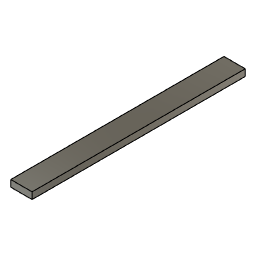
Assembly (no drawer) (Autodesk Fusion 360 archive; units mm, degrees)
design "Rail (2x)"
Autodesk Fusion 360 part; units mm, degrees
sketch "Sketch1" plane through (0, 0, 0) normal (0, 0, 1) x (1, 0, 0)
  line L0 (0, 0) -> (10.16, 0)
  line L1 (10.16, 0) -> (10.16, 101.6)
  line L2 (10.16, 101.6) -> (0, 101.6)
  line L3 (0, 101.6) -> (0, 0)
  dimension "d1" = 10.16
  dimension "d2" = 101.6
  constraint coincident L0.start L3.end
  constraint horizontal L0
  constraint perpendicular L0 L1
  constraint perpendicular L1 L2
  constraint perpendicular L0 L3
  measures "d1" distance of L0.start L0.end
  measures "d2" distance of L0.end L1.end
extrude "Extrude1" add sketch "Sketch1" along normal blind 3.175

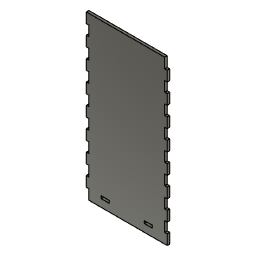
design "Dice Tower (Back)"
Autodesk Fusion 360 part; units mm, degrees
sketch "Sketch1" plane through (0, 0, 0) normal (0, 1, 0) x (1, 0, 0)
  line L0 (3.175, -50.8) -> (3.175, -38.1)
  line L1 (3.175, -38.1) -> (3.175, -25.4)
  line L2 (6.35, -12.7) -> (3.175, -12.7)
  line L3 (3.175, -63.5) -> (6.35, -63.5)
  line L4 (3.175, -76.2) -> (3.175, -63.5)
  line L5 (6.35, -25.4) -> (3.175, -25.4)
  line L6 (3.175, -88.9) -> (3.175, -76.2)
  line L7 (6.35, -25.4) -> (6.35, -38.1)
  line L8 (6.35, -38.1) -> (3.175, -38.1)
  line L9 (3.175, -12.7) -> (3.175, 0)
  line L10 (3.175, -60.2676) -> (2.1543, -60.2676)
  line L11 (3.175, 0) -> (3.175, -59.055)
  line L12 (6.35, 0) -> (3.175, 0)
  line L13 (3.175, -25.4) -> (3.175, -12.7)
  line L14 (3.175, -101.6) -> (3.175, -88.9)
  line L15 (3.175, -76.2) -> (6.35, -76.2)
  line L16 (-95.25, -25.4) -> (-95.25, -12.7)
  line L17 (-92.075, -139.7) -> (-95.25, -139.7)
  line L18 (3.175, 0) -> (3.175, -203.2)
  line L19 (-92.075, -50.8) -> (-95.25, -50.8)
  line L20 (3.175, -50.8) -> (6.35, -50.8)
  line L21 (6.35, 0) -> (-4.7498, 0)
  line L22 (3.175, -88.9) -> (6.35, -88.9)
  line L23 (-92.075, -38.1) -> (-92.075, -25.4)
  line L24 (-92.075, -127) -> (-92.075, -114.3)
  line L25 (-95.25, 0) -> (6.35, 0)
  line L26 (-92.075, -203.2) -> (-92.075, -190.5)
  line L27 (3.175, -63.5) -> (3.175, -50.8)
  line L28 (6.35, -50.8) -> (6.35, -63.5)
  line L29 (-92.075, 0) -> (-92.075, -203.2)
  line L30 (6.35, -76.2) -> (6.35, -88.9)
  line L31 (-92.075, -95.25) -> (-92.075, -88.9)
  line L32 (6.35, 0) -> (-5.715, 0)
  line L33 (-95.25, 0) -> (-79.375, 0)
  line L34 (-92.075, -25.4) -> (-95.25, -25.4)
  line L35 (-92.075, -76.2) -> (-92.075, -63.5)
  line L36 (-4.7498, 0) -> (0.3302, 0)
  line L37 (6.35, 0) -> (6.35, -12.7)
  line L38 (6.35, -101.6) -> (3.175, -101.6)
  line L39 (-92.075, -177.8) -> (-95.25, -177.8)
  line L40 (-84.1502, 0) -> (-89.2302, 0)
  line L41 (-92.075, -139.7) -> (-92.075, -127)
  line L42 (-89.5189, -92.8088) -> (-89.7576, -92.8956)
  line L43 (-95.25, -101.6) -> (-95.25, -88.9)
  line L44 (6.35, -177.8) -> (6.35, -190.5)
  line L45 (6.35, -152.4) -> (6.35, -165.1)
  line L46 (3.175, -203.2) -> (3.175, -190.5)
  line L47 (3.175, -190.5) -> (3.175, -177.8)
  line L48 (-92.075, -63.5) -> (-95.25, -63.5)
  line L49 (-92.075, -25.4) -> (-92.075, -12.7)
  line L50 (-92.075, -190.5) -> (-95.25, -190.5)
  line L51 (-92.075, -12.7) -> (-95.25, -12.7)
  line L52 (3.175, -203.2) -> (-95.25, -203.2)
  line L53 (-92.075, -177.8) -> (-92.075, -165.1)
  line L54 (-92.075, -101.6) -> (-92.075, -95.25)
  line L55 (-92.075, -76.2) -> (-95.25, -76.2)
  line L56 (-95.25, -76.2) -> (-95.25, -63.5)
  line L57 (3.175, -114.3) -> (6.35, -114.3)
  line L58 (-95.25, -203.2) -> (-95.25, -190.5)
  line L59 (-92.075, -63.5) -> (-92.075, -50.8)
  line L60 (-92.075, -50.8) -> (-92.075, -38.1)
  line L61 (-92.075, -152.4) -> (-95.25, -152.4)
  line L62 (-92.075, -88.9) -> (-95.25, -88.9)
  line L63 (-92.075, -152.4) -> (-92.075, -139.7)
  line L64 (-95.25, -203.2) -> (-92.075, -203.2)
  line L65 (6.35, -152.4) -> (3.175, -152.4)
  line L66 (-92.075, -165.1) -> (-92.075, -152.4)
  line L67 (-92.075, -203.2) -> (-92.075, -177.8)
  line L68 (-92.075, -165.1) -> (-95.25, -165.1)
  line L69 (-92.075, -114.3) -> (-95.25, -114.3)
  line L70 (6.35, -101.6) -> (6.35, -114.3)
  line L71 (-95.25, -127) -> (-95.25, -114.3)
  line L72 (-92.075, -114.3) -> (-92.075, -101.6)
  line L73 (6.35, -139.7) -> (6.35, -127)
  line L74 (6.35, -127) -> (6.35, -139.7)
  line L75 (3.175, -177.8) -> (6.35, -177.8)
  line L76 (3.175, -165.1) -> (6.35, -165.1)
  line L77 (-92.075, -38.1) -> (-95.25, -38.1)
  line L78 (6.35, -114.3) -> (6.35, -101.6)
  line L79 (-95.25, 0) -> (-84.1502, 0)
  line L80 (-92.075, -127) -> (-95.25, -127)
  line L81 (3.175, -152.4) -> (3.175, -139.7)
  line L82 (-95.25, -177.8) -> (-95.25, -165.1)
  line L83 (6.35, -165.1) -> (6.35, -152.4)
  line L84 (-92.075, -101.6) -> (-95.25, -101.6)
  line L85 (3.175, -139.7) -> (6.35, -139.7)
  line L86 (-95.25, 0) -> (-92.075, 0)
  line L87 (-95.25, -152.4) -> (-95.25, -139.7)
  line L88 (3.175, -127) -> (3.175, -114.3)
  line L89 (6.35, -127) -> (3.175, -127)
  line L90 (3.175, -190.5) -> (6.35, -190.5)
  line L91 (-92.075, -88.9) -> (-92.075, -76.2)
  line L92 (-95.25, 0) -> (-93.6625, 0)
  line L93 (-92.075, -190.5) -> (-92.075, -177.8)
  line L94 (3.175, -177.8) -> (3.175, -165.1)
  line L95 (-95.25, -50.8) -> (-95.25, -38.1)
  point P0 (6.35, 0)
  point P1 (6.35, 0)
  dimension "d9" = 11.0998
  dimension "d10" = 11.0998
  dimension "d14" = 5.08
  dimension "d15" = 5.08
  dimension "d27" = 3.175
  dimension "d28" = 3.175
  dimension "d40" = 3.175
  dimension "d41" = 3.175
  dimension "d42" = 12.7
  dimension "d43" = 12.7
  dimension "d44" = 12.7
  dimension "d45" = 12.7
  dimension "d46" = 12.7
  dimension "d47" = 12.7
  dimension "d48" = 12.7
  dimension "d49" = 12.7
  dimension "d50" = 6.35
  dimension "d52" = 12.7
  dimension "d53" = 12.7
  dimension "d54" = 12.7
  dimension "d55" = 12.7
  dimension "d56" = 12.7
  dimension "d57" = 12.7
  constraint coincident P1 P0
  constraint perpendicular L37 L52
  constraint perpendicular L52 L58
  constraint perpendicular L25 L37
  constraint perpendicular L32 L37
  constraint perpendicular L33 L58
  constraint perpendicular L58 L92
  constraint coincident L40.start L25
  constraint perpendicular L21 L37
  constraint perpendicular L37 L90
  constraint perpendicular L47 L90
  constraint coincident L44.start L37
  constraint perpendicular L37 L75
  constraint perpendicular L75 L94
  constraint perpendicular L37 L76
  constraint collinear L37 L44
  constraint perpendicular L76 L83
  constraint perpendicular L65 L83
  constraint parallel L12 L32
  constraint perpendicular L18 L52
  constraint perpendicular L65 L81
  constraint coincident L88.start L18
  constraint perpendicular L18 L89
  constraint perpendicular L88 L89
  constraint perpendicular L57 L88
  constraint perpendicular L18 L38
  constraint perpendicular L14 L38
  constraint parallel L0 L1
  constraint parallel L13 L18
  constraint coincident L15.end L37
  constraint coincident L20.end L37
  constraint coincident L5.start L37
  constraint collinear L37 L45
  constraint collinear L37 L74
  constraint collinear L37 L70
  constraint collinear L30 L37
  constraint collinear L28 L37
  constraint collinear L7 L37
  constraint perpendicular L58 L64
  constraint perpendicular L58 L86
  constraint perpendicular L26 L52
  constraint perpendicular L50 L58
  constraint perpendicular L50 L93
  constraint coincident L39.end L58
  constraint perpendicular L39 L58
  constraint perpendicular L39 L53
  constraint coincident L68.end L58
  constraint perpendicular L58 L68
  constraint perpendicular L66 L68
  constraint coincident L61.end L58
  constraint perpendicular L58 L61
  constraint perpendicular L61 L63
  constraint coincident L17.end L58
  constraint perpendicular L17 L58
  constraint perpendicular L17 L41
  constraint coincident L71.start L58
  constraint perpendicular L58 L80
  constraint perpendicular L24 L80
  constraint coincident L69.end L58
  constraint perpendicular L58 L69
  constraint perpendicular L69 L72
  constraint perpendicular L58 L84
  constraint perpendicular L54 L84
  constraint parallel L29 L31
  constraint coincident L43.end L58
  constraint perpendicular L58 L62
  constraint perpendicular L62 L91
  constraint coincident L55.end L58
  constraint perpendicular L55 L58
  constraint perpendicular L35 L55
  constraint coincident L48.end L58
  constraint perpendicular L48 L58
  constraint perpendicular L48 L59
  constraint coincident L19.end L58
  constraint perpendicular L19 L58
  constraint perpendicular L19 L60
  constraint coincident L77.end L58
  constraint perpendicular L58 L77
  constraint perpendicular L23 L77
  constraint perpendicular L23 L34
  constraint perpendicular L34 L49
  constraint perpendicular L49 L51
  constraint collinear L58 L82
  constraint coincident L43.start L58
  constraint collinear L82 L87
  constraint collinear L71 L87
  constraint collinear L43 L71
  constraint collinear L43 L56
  constraint collinear L56 L95
  constraint collinear L16 L95
  constraint coincident L11.end L27
  constraint coincident L10.start L27
  measures "d9" distance of L40.start L25.start
  measures "d10" distance of P1 L21.end
  measures "d14" distance of L36.end L21.end
  measures "d15" distance of L40.start L40.end
  measures "d27" distance of L65.end L45.start
  measures "d28" distance of P1 L9.end
  measures "d40" distance of L52.end L26.start
  measures "d41" distance of L25.start L29.start
  measures "d42" distance of L26.end L26.start
  measures "d43" distance of L39.start L26.end
  measures "d44" distance of L39.start L53.end
  measures "d45" distance of L61.start L53.end
  measures "d46" distance of L61.start L17.start
  measures "d47" distance of L24.start L17.start
  measures "d48" distance of L24.start L24.end
  measures "d49" distance of L54.start L24.end
  measures "d50" distance of L54.start L31.start
  measures "d52" distance of L35.start L31.end
  measures "d53" distance of L35.start L35.end
  measures "d54" distance of L19.start L35.end
  measures "d55" distance of L23.start L19.start
  measures "d56" distance of L23.end L23.start
  measures "d57" distance of L49.end L23.end
extrude "Extrude1" add sketch "Sketch1" along normal blind 3.175
sketch "Sketch2" plane through (0, 0, 0) normal (0, -1, 0) x (1, 0, 0)
  line L0 (-95.25, 63.5) -> (-92.075, 63.5)
  line L1 (-92.075, 63.5) -> (-92.075, 50.8)
  line L2 (-92.075, 50.8) -> (-95.25, 50.8)
  line L3 (-95.25, 50.8) -> (-95.25, 38.1)
  line L4 (-95.25, 38.1) -> (-92.075, 38.1)
  line L5 (-92.075, 38.1) -> (-92.075, 25.4)
  line L6 (-92.075, 25.4) -> (-95.25, 25.4)
  line L7 (-95.25, 25.4) -> (-95.25, 12.7)
  line L8 (-95.25, 12.7) -> (-92.075, 12.7)
  line L9 (-92.075, 12.7) -> (-92.075, 0)
  line L10 (-92.075, 0) -> (6.35, 0)
  line L11 (6.35, 0) -> (6.35, 12.7)
  line L12 (6.35, 12.7) -> (3.175, 12.7)
  line L13 (3.175, 12.7) -> (3.175, 25.4)
  line L14 (3.175, 25.4) -> (6.35, 25.4)
  line L15 (6.35, 25.4) -> (6.35, 38.1)
  line L16 (6.35, 38.1) -> (3.175, 38.1)
  line L17 (3.175, 38.1) -> (3.175, 50.8)
  line L18 (3.175, 50.8) -> (6.35, 50.8)
  line L19 (6.35, 50.8) -> (6.35, 63.5)
  line L20 (6.35, 63.5) -> (3.175, 63.5)
  line L21 (3.175, 63.5) -> (3.175, 76.2)
  line L22 (3.175, 76.2) -> (6.35, 76.2)
  line L23 (6.35, 76.2) -> (6.35, 88.9)
  line L24 (6.35, 88.9) -> (3.175, 88.9)
  line L25 (3.175, 88.9) -> (3.175, 101.6)
  line L26 (3.175, 101.6) -> (6.35, 101.6)
  line L27 (6.35, 101.6) -> (6.35, 114.3)
  line L28 (6.35, 114.3) -> (3.175, 114.3)
  line L29 (3.175, 114.3) -> (3.175, 127)
  line L30 (3.175, 127) -> (6.35, 127)
  line L31 (6.35, 127) -> (6.35, 139.7)
  line L32 (6.35, 139.7) -> (3.175, 139.7)
  line L33 (3.175, 139.7) -> (3.175, 152.4)
  line L34 (3.175, 152.4) -> (6.35, 152.4)
  line L35 (6.35, 152.4) -> (6.35, 165.1)
  line L36 (6.35, 165.1) -> (3.175, 165.1)
  line L37 (3.175, 165.1) -> (3.175, 177.8)
  line L38 (3.175, 177.8) -> (6.35, 177.8)
  line L39 (6.35, 177.8) -> (6.35, 190.5)
  line L40 (6.35, 190.5) -> (3.175, 190.5)
  line L41 (3.175, 190.5) -> (3.175, 203.2)
  line L42 (3.175, 203.2) -> (-95.25, 203.2)
  line L43 (-95.25, 203.2) -> (-95.25, 190.5)
  line L44 (-95.25, 190.5) -> (-92.075, 190.5)
  line L45 (-92.075, 190.5) -> (-92.075, 177.8)
  line L46 (-92.075, 177.8) -> (-95.25, 177.8)
  line L47 (-95.25, 177.8) -> (-95.25, 165.1)
  line L48 (-95.25, 165.1) -> (-92.075, 165.1)
  line L49 (-92.075, 165.1) -> (-92.075, 152.4)
  line L50 (-92.075, 152.4) -> (-95.25, 152.4)
  line L51 (-95.25, 152.4) -> (-95.25, 139.7)
  line L52 (-95.25, 139.7) -> (-92.075, 139.7)
  line L53 (-92.075, 139.7) -> (-92.075, 127)
  line L54 (-92.075, 127) -> (-95.25, 127)
  line L55 (-95.25, 127) -> (-95.25, 114.3)
  line L56 (-95.25, 114.3) -> (-92.075, 114.3)
  line L57 (-92.075, 114.3) -> (-92.075, 101.6)
  line L58 (-92.075, 101.6) -> (-95.25, 101.6)
  line L59 (-95.25, 101.6) -> (-95.25, 88.9)
  line L60 (-95.25, 88.9) -> (-92.075, 88.9)
  line L61 (-92.075, 88.9) -> (-92.075, 76.2)
  line L62 (-92.075, 76.2) -> (-95.25, 76.2)
  line L63 (-95.25, 76.2) -> (-95.25, 63.5)
  line L64 (6.35, 0) -> (-12.3698, 0)
  line L65 (-12.3698, 0) -> (-12.3698, 9.525)
  line L66 (-92.075, 0) -> (-76.5302, 0)
  line L67 (-76.5302, 0) -> (-76.5302, 9.525)
  line L68 (-76.5302, 9.525) -> (-66.3702, 9.525)
  line L69 (-66.3702, 9.525) -> (-66.3702, 12.7)
  line L70 (-66.3702, 12.7) -> (-76.5302, 12.7)
  line L71 (-76.5302, 12.7) -> (-76.5302, 9.525)
  line L72 (-12.3698, 9.525) -> (-22.5298, 9.525)
  line L73 (-22.5298, 9.525) -> (-22.5298, 12.7)
  line L74 (-22.5298, 12.7) -> (-12.3698, 12.7)
  line L75 (-12.3698, 12.7) -> (-12.3698, 9.525)
  dimension "d105" = 18.7198
  dimension "d106" = 9.525
  dimension "d107" = 15.5448
  dimension "d108" = 9.525
  dimension "d109" = 10.16
  dimension "d110" = 3.175
  dimension "d111" = 10.16
  dimension "d112" = 10.16
  dimension "d113" = 10.16
  constraint coincident L10.end L11.start
  constraint perpendicular L11 L64
  constraint perpendicular L64 L65
  constraint coincident L9.end L10.start
  constraint perpendicular L9 L66
  constraint perpendicular L66 L67
  constraint perpendicular L67 L68
  constraint perpendicular L68 L69
  constraint perpendicular L69 L70
  constraint perpendicular L65 L72
  constraint perpendicular L72 L73
  constraint perpendicular L73 L74
  measures "d105" distance of L10.end L64.end
  measures "d106" distance of L64.end L65.end
  measures "d107" distance of L9.end L66.end
  measures "d108" distance of L66.end L67.end
  measures "d109" distance of L67.end L68.end
  measures "d110" distance of L68.end L69.end
  measures "d111" distance of L69.end L70.end
  measures "d112" distance of L65.end L72.end
  measures "d113" distance of L73.end L74.end
extrude "Extrude2" cut sketch "Sketch2" against normal blind 20.32 contours L68 L69 L70 L71 | L72 L73 L74 L75
equation "d9 = 0.5 in - 0.063 in"

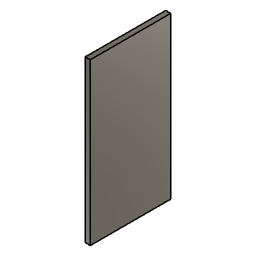
design "Ramp (Top Ramp x2)"
Autodesk Fusion 360 part; units mm, degrees
sketch "Sketch1" plane through (0, 0, 0) normal (1, 0, 0) x (0, 1, 0)
  line L0 (0, 0) -> (50.8, 0)
  line L1 (50.8, 0) -> (50.8, 101.6)
  line L2 (50.8, 101.6) -> (0, 101.6)
  line L3 (0, 101.6) -> (0, 0)
  dimension "d1" = 50.8
  dimension "d2" = 101.6
  constraint coincident L0.start L3.end
  constraint horizontal L0
  constraint perpendicular L0 L1
  constraint perpendicular L1 L2
  constraint perpendicular L2 L3
  measures "d1" distance of L0.start L0.end
  measures "d2" distance of L0.end L1.end
extrude "Extrude1" add sketch "Sketch1" along normal blind 3.175

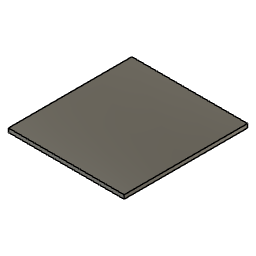
design "Ramp (Bottem Ramp 1x)"
Autodesk Fusion 360 part; units mm, degrees
sketch "Sketch1" plane through (0, 0, 0) normal (0, 0, 1) x (1, 0, 0)
  line L0 (0, 0) -> (95.25, 0)
  line L1 (95.25, 0) -> (95.25, 101.6)
  line L2 (95.25, 101.6) -> (0, 101.6)
  line L3 (0, 101.6) -> (0, 0)
  dimension "d1" = 95.25
  dimension "d2" = 101.6
  dimension "d3" = 95.25
  constraint coincident L0.start L3.end
  constraint horizontal L0
  constraint perpendicular L0 L1
  constraint perpendicular L1 L2
  measures "d1" distance of L0.start L0.end
  measures "d2" distance of L0.end L1.end
  measures "d3" distance of L1.end L2.end
extrude "Extrude1" add sketch "Sketch1" along normal blind 3.175

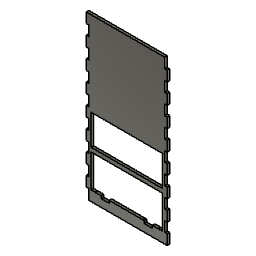
design "Dice Tower (FRONT)"
Autodesk Fusion 360 part; units mm, degrees
sketch "Sketch2" plane through (0, 0, 0) normal (0, 0, 1) x (1, 0, 0)
sketch "Sketch3" plane through (0, 0, 0) normal (0, 1, 0) x (1, 0, 0)
  line L0 (85.725, 0) -> (101.6, 0)
  line L1 (88.9, -50.8) -> (85.725, -50.8)
  line L2 (187.325, -12.7) -> (184.15, -12.7)
  line L3 (104.4448, -12.7) -> (104.4448, -9.525)
  line L4 (88.9, -12.7) -> (85.725, -12.7)
  line L5 (85.725, -25.4) -> (85.725, -12.7)
  line L6 (91.7448, -12.7) -> (104.4448, -12.7)
  line L7 (88.9, -63.5) -> (88.9, -50.8)
  line L8 (181.3052, -12.7) -> (168.6052, -12.7)
  line L9 (88.9, -76.2) -> (88.9, -63.5)
  line L10 (181.3052, -53.975) -> (91.7448, -53.975)
  line L11 (85.725, 0) -> (87.3125, 0)
  line L12 (91.7448, 0) -> (91.7448, -12.7)
  line L13 (88.9, -50.8) -> (88.9, -38.1)
  line L14 (88.9, -25.4) -> (88.9, -12.7)
  line L15 (176.2252, 0) -> (181.3052, 0)
  line L16 (187.325, -38.1) -> (184.15, -38.1)
  line L17 (158.4452, -12.7) -> (156.5402, -12.7)
  line L18 (96.8248, -12.7) -> (104.4448, -12.7)
  line L19 (168.6052, -12.7) -> (176.2252, -12.7)
  line L20 (91.7448, -12.7) -> (96.8248, -12.7)
  line L21 (88.9, -38.1) -> (88.9, -25.4)
  line L22 (168.6052, -12.7) -> (168.6052, -9.525)
  line L23 (96.8248, 0) -> (91.7448, 0)
  line L24 (187.325, -25.4) -> (184.15, -25.4)
  line L25 (88.9, -25.4) -> (85.725, -25.4)
  line L26 (114.6048, -12.7) -> (156.5402, -12.7)
  line L27 (158.4452, -9.525) -> (158.4452, -12.7)
  line L28 (114.6048, -9.525) -> (114.6048, -12.7)
  line L29 (187.325, 0) -> (187.325, -12.7)
  line L30 (181.3052, -12.7) -> (176.2252, -12.7)
  line L31 (187.325, 0) -> (184.15, 0)
  line L32 (85.725, 0) -> (96.8248, 0)
  line L33 (187.325, 0) -> (176.2252, 0)
  line L34 (184.15, -12.7) -> (184.15, 0)
  line L35 (184.15, -25.4) -> (184.15, -12.7)
  line L36 (88.9, -139.7) -> (85.725, -139.7)
  line L37 (88.9, -101.6) -> (88.9, -95.25)
  line L38 (88.9, -127) -> (85.725, -127)
  line L39 (88.9, -95.25) -> (88.9, -88.9)
  line L40 (184.15, -101.6) -> (184.15, -88.9)
  line L41 (88.9, -114.3) -> (88.9, -101.6)
  line L42 (187.325, -101.6) -> (187.325, -114.3)
  line L43 (184.15, -127) -> (184.15, -114.3)
  line L44 (88.9, -127) -> (88.9, -114.3)
  line L45 (187.325, -101.6) -> (184.15, -101.6)
  line L46 (187.325, -139.7) -> (187.325, -127)
  line L47 (184.15, -139.7) -> (187.325, -139.7)
  line L48 (88.9, -114.3) -> (85.725, -114.3)
  line L49 (88.9, -139.7) -> (88.9, -127)
  line L50 (187.325, -114.3) -> (187.325, -101.6)
  line L51 (187.325, -127) -> (184.15, -127)
  line L52 (88.9, -88.9) -> (85.725, -88.9)
  line L53 (91.7448, -97.155) -> (181.3052, -97.155)
  line L54 (85.725, -101.6) -> (85.725, -88.9)
  line L55 (88.9, -101.6) -> (85.725, -101.6)
  line L56 (187.325, -127) -> (187.325, -139.7)
  line L57 (184.15, -88.9) -> (187.325, -88.9)
  line L58 (184.15, -114.3) -> (187.325, -114.3)
  line L59 (85.725, -127) -> (85.725, -114.3)
  line L60 (184.15, 0) -> (184.15, -203.2)
  line L61 (85.725, -203.2) -> (88.9, -203.2)
  line L62 (88.9, 0) -> (88.9, -203.2)
  line L63 (88.9, -165.1) -> (88.9, -152.4)
  line L64 (187.325, -152.4) -> (187.325, -165.1)
  line L65 (184.15, -203.2) -> (184.15, -190.5)
  line L66 (184.15, -152.4) -> (184.15, -139.7)
  line L67 (88.9, -203.2) -> (88.9, -190.5)
  line L68 (85.725, -152.4) -> (85.725, -139.7)
  line L69 (88.9, -165.1) -> (85.725, -165.1)
  line L70 (88.9, -190.5) -> (85.725, -190.5)
  line L71 (88.9, -177.8) -> (85.725, -177.8)
  line L72 (184.15, -177.8) -> (187.325, -177.8)
  line L73 (184.15, -190.5) -> (184.15, -177.8)
  line L74 (88.9, -152.4) -> (88.9, -139.7)
  line L75 (184.15, -165.1) -> (187.325, -165.1)
  line L76 (187.325, -177.8) -> (187.325, -190.5)
  line L77 (88.9, -152.4) -> (85.725, -152.4)
  line L78 (187.325, -152.4) -> (184.15, -152.4)
  line L79 (184.15, -190.5) -> (187.325, -190.5)
  line L80 (184.15, -76.2) -> (187.325, -76.2)
  line L81 (181.3052, 0) -> (181.3052, -12.7)
  line L82 (91.7448, -59.055) -> (181.3052, -59.055)
  line L83 (187.325, -165.1) -> (187.325, -152.4)
  line L84 (91.7448, -59.055) -> (91.7448, -97.155)
  line L85 (88.9, -63.5) -> (85.725, -63.5)
  line L86 (184.15, -177.8) -> (184.15, -165.1)
  line L87 (184.15, -50.8) -> (184.15, -38.1)
  line L88 (85.725, 0) -> (187.325, 0)
  line L89 (184.15, -63.5) -> (187.325, -63.5)
  line L90 (187.325, -25.4) -> (187.325, -38.1)
  line L91 (187.325, 0) -> (175.26, 0)
  line L92 (184.15, -76.2) -> (184.15, -63.5)
  line L93 (181.3052, -59.055) -> (181.3052, -97.155)
  line L94 (187.325, -50.8) -> (187.325, -63.5)
  line L95 (168.6052, -9.525) -> (158.4452, -9.525)
  line L96 (184.15, -38.1) -> (184.15, -25.4)
  line L97 (85.725, -76.2) -> (85.725, -63.5)
  line L98 (85.725, -177.8) -> (85.725, -165.1)
  line L99 (91.7448, -12.7) -> (91.7448, -53.975)
  line L100 (85.725, -50.8) -> (85.725, -38.1)
  line L101 (104.4448, -9.525) -> (114.6048, -9.525)
  line L102 (184.15, -50.8) -> (187.325, -50.8)
  line L103 (88.9, -177.8) -> (88.9, -165.1)
  line L104 (181.3052, -12.7) -> (181.3052, -53.975)
  line L105 (187.325, -76.2) -> (187.325, -88.9)
  line L106 (88.9, -190.5) -> (88.9, -177.8)
  line L107 (184.15, -88.9) -> (184.15, -76.2)
  line L108 (184.15, -203.2) -> (85.725, -203.2)
  line L109 (88.9, -76.2) -> (85.725, -76.2)
  line L110 (88.9, -88.9) -> (88.9, -76.2)
  line L111 (88.9, -38.1) -> (85.725, -38.1)
  line L112 (85.725, 0) -> (88.9, 0)
  line L113 (91.7448, -53.975) -> (91.7448, -59.055)
  line L114 (85.725, -203.2) -> (85.725, -190.5)
  line L115 (184.15, -63.5) -> (184.15, -50.8)
  point P0 (187.325, 0)
  dimension "d68" = 11.0998
  dimension "d69" = 11.0998
  dimension "d70" = 12.7
  dimension "d71" = 12.7
  dimension "d72" = 5.08
  dimension "d73" = 5.08
  dimension "d74" = 41.275
  dimension "d75" = 5.08
  dimension "d76" = 5.08
  dimension "d77" = 38.1
  dimension "d78" = 3.175
  dimension "d79" = 3.175
  dimension "d80" = 3.175
  dimension "d81" = 3.175
  dimension "d82" = 12.7
  dimension "d83" = 12.7
  dimension "d84" = 12.7
  dimension "d85" = 12.7
  dimension "d86" = 12.7
  dimension "d87" = 12.7
  dimension "d88" = 12.7
  dimension "d89" = 12.7
  dimension "d90" = 6.35
  dimension "d91" = 6.35
  dimension "d92" = 12.7
  dimension "d93" = 12.7
  dimension "d94" = 12.7
  dimension "d95" = 12.7
  dimension "d96" = 12.7
  dimension "d97" = 12.7
  dimension "d98" = 12.7
  dimension "d99" = 12.7
  dimension "d100" = 3.175
  dimension "d101" = 10.16
  dimension "d102" = 3.175
  dimension "d103" = 10.16
  constraint coincident P0 L29.start
  constraint perpendicular L29 L108
  constraint perpendicular L108 L114
  constraint perpendicular L29 L88
  constraint perpendicular L29 L91
  constraint perpendicular L0 L114
  constraint perpendicular L11 L114
  constraint coincident L23.start L88
  constraint perpendicular L29 L33
  constraint perpendicular L12 L23
  constraint perpendicular L81 L91
  constraint perpendicular L20 L99
  constraint perpendicular L30 L104
  constraint perpendicular L10 L113
  constraint perpendicular L82 L93
  constraint perpendicular L82 L84
  constraint perpendicular L29 L79
  constraint perpendicular L73 L79
  constraint coincident L72.end L29
  constraint perpendicular L29 L72
  constraint perpendicular L72 L86
  constraint perpendicular L29 L75
  constraint collinear L29 L76
  constraint perpendicular L75 L83
  constraint perpendicular L78 L83
  constraint parallel L31 L91
  constraint perpendicular L60 L108
  constraint perpendicular L66 L78
  constraint perpendicular L29 L47
  constraint perpendicular L46 L47
  constraint coincident L43.start L60
  constraint perpendicular L51 L60
  constraint perpendicular L43 L51
  constraint perpendicular L43 L58
  constraint perpendicular L50 L58
  constraint midpoint L40.start L60
  constraint perpendicular L45 L60
  constraint perpendicular L40 L45
  constraint parallel L60 L107
  constraint parallel L60 L92
  constraint parallel L60 L115
  constraint parallel L60 L87
  constraint parallel L87 L96
  constraint parallel L35 L60
  constraint perpendicular L29 L57
  constraint coincident L80.end L29
  constraint perpendicular L29 L80
  constraint perpendicular L29 L89
  constraint coincident L94.start L29
  constraint perpendicular L29 L102
  constraint coincident L24.start L29
  constraint collinear L29 L64
  constraint collinear L29 L56
  constraint collinear L29 L42
  constraint collinear L29 L105
  constraint collinear L29 L94
  constraint collinear L29 L90
  constraint perpendicular L61 L114
  constraint perpendicular L112 L114
  constraint perpendicular L67 L108
  constraint perpendicular L70 L114
  constraint perpendicular L70 L106
  constraint coincident L71.end L114
  constraint perpendicular L71 L114
  constraint perpendicular L71 L103
  constraint coincident L69.end L114
  constraint perpendicular L69 L114
  constraint perpendicular L63 L69
  constraint coincident L68.start L114
  constraint perpendicular L77 L114
  constraint perpendicular L74 L77
  constraint coincident L36.end L114
  constraint perpendicular L36 L114
  constraint perpendicular L36 L49
  constraint coincident L38.end L114
  constraint perpendicular L38 L114
  constraint perpendicular L38 L44
  constraint coincident L48.end L114
  constraint perpendicular L48 L114
  constraint perpendicular L41 L48
  constraint perpendicular L55 L114
  constraint perpendicular L37 L55
  constraint parallel L39 L62
  constraint coincident L52.end L114
  constraint perpendicular L52 L114
  constraint perpendicular L52 L110
  constraint coincident L97.start L114
  constraint perpendicular L109 L114
  constraint perpendicular L9 L109
  constraint coincident L85.end L114
  constraint perpendicular L85 L114
  constraint perpendicular L7 L85
  constraint coincident L1.end L114
  constraint perpendicular L1 L114
  constraint perpendicular L1 L13
  constraint coincident L100.end L114
  constraint perpendicular L111 L114
  constraint perpendicular L21 L111
  constraint perpendicular L21 L25
  constraint perpendicular L14 L25
  constraint perpendicular L4 L14
  constraint collinear L98 L114
  constraint coincident L54.start L114
  constraint collinear L68 L98
  constraint collinear L59 L68
  constraint collinear L54 L59
  constraint collinear L54 L97
  constraint collinear L97 L100
  constraint collinear L5 L100
  constraint perpendicular L8 L81
  constraint collinear L18 L19
  constraint perpendicular L6 L12
  constraint perpendicular L3 L18
  constraint perpendicular L3 L101
  constraint perpendicular L28 L101
  constraint collinear L18 L26
  constraint perpendicular L22 L95
  constraint perpendicular L27 L95
  measures "d68" distance of L0.start L23.start
  measures "d69" distance of P0 L15.start
  measures "d70" distance of L19.end L15.start
  measures "d71" distance of L23.start L18.start
  measures "d72" distance of L15.end L15.start
  measures "d73" distance of L23.start L12.start
  measures "d74" distance of L10.end L6.start
  measures "d75" distance of L10.start L82.end
  measures "d76" distance of L82.start L10.end
  measures "d77" distance of L53.start L82.start
  measures "d78" distance of L64.start L66.start
  measures "d79" distance of L31.end P0
  measures "d80" distance of L61.start L61.end
  measures "d81" distance of L0.start L62.start
  measures "d82" distance of L61.end L67.end
  measures "d83" distance of L71.start L67.end
  measures "d84" distance of L71.start L63.start
  measures "d85" distance of L63.end L63.start
  measures "d86" distance of L63.end L36.start
  measures "d87" distance of L38.start L36.start
  measures "d88" distance of L41.start L38.start
  measures "d89" distance of L37.start L41.start
  measures "d90" distance of L37.end L37.start
  measures "d91" distance of L37.end L39.end
  measures "d92" distance of L9.start L39.end
  measures "d93" distance of L9.start L7.start
  measures "d94" distance of L1.start L7.start
  measures "d95" distance of L13.end L1.start
  measures "d96" distance of L13.end L14.start
  measures "d97" distance of L4.start L14.start
  measures "d98" distance of L8.end L8.start
  measures "d99" distance of L3.start L6.start
  measures "d100" distance of L3.end L3.start
  measures "d101" distance of L28.start L3.end
  measures "d102" distance of L8.end L22.end
  measures "d103" distance of L27.start L22.end
extrude "Extrude1" add sketch "Sketch3" along normal blind 3.175 contours L0 L7 L9 L10 L12 L13 L14 L21 L32 L33 L34 L35 L37 L39 L40 L41 L43 L44 L49 L60 L62 L63 L65 L66 L67 L73 L74 L81 L86 L87 L88 L91 L92 L96 L99 L103 L104 L106 L107 L108 L110 L115 | L0 L3 L6 L8 L12 L15 L17 L18 L19 L20 L22 L23 L26 L27 L28 L30 L32 L33 L81 L88 L91 L95 L101 | L4 L5 L14 L25 L62 | L1 L13 L62 L100 L111 | L9 L62 L85 L97 L109 | L2 L29 L31 L33 L34 L60 L88 L91 | L37 L39 L52 L54 L55 L62 | L16 L24 L60 L90 L96 | L38 L44 L48 L59 L62 | L60 L89 L94 L102 L115 | L36 L62 L68 L74 L77 | L57 L60 L80 L105 L107 | L62 L69 L71 L98 L103 | L42 L45 L50 L58 L60 | L61 L62 L67 L70 L108 L114 | L46 L47 L51 L56 L60 | L60 L64 L75 L78 L83 | L60 L72 L73 L76 L79
equation "d68 = 0.5 in - 0.063 in"
equation "d74 = 1.5 in + 0.125 in"

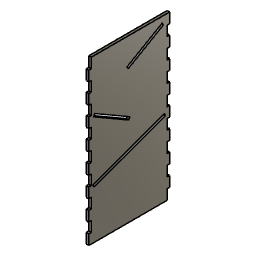
design "Dice Tower (Right Side)"
Autodesk Fusion 360 part; units mm, degrees
sketch "Sketch1" plane through (0, 0, 0) normal (1, 0, 0) x (0, 1, 0)
  line L0 (98.425, 139.7) -> (101.6, 139.7)
  line L1 (0, 101.6) -> (0, 114.3)
  line L2 (0, 127) -> (0, 139.7)
  line L3 (98.425, 114.3) -> (101.6, 114.3)
  line L4 (0, 127) -> (3.175, 127)
  line L5 (101.6, 101.6) -> (101.6, 88.9)
  line L6 (0, 101.6) -> (3.175, 101.6)
  line L7 (98.425, 0) -> (98.425, 203.2)
  line L8 (98.425, 114.3) -> (98.425, 101.6)
  line L9 (98.425, 88.9) -> (101.6, 88.9)
  line L10 (101.6, 0) -> (100.0125, 0)
  line L11 (98.425, 127) -> (101.6, 127)
  line L12 (98.425, 101.6) -> (101.6, 101.6)
  line L13 (98.425, 95.25) -> (98.425, 88.9)
  line L14 (3.175, 0) -> (3.175, 203.2)
  line L15 (101.6, 127) -> (101.6, 114.3)
  line L16 (3.175, 127) -> (3.175, 114.3)
  line L17 (3.175, 88.9) -> (0, 88.9)
  line L18 (98.425, 139.7) -> (98.425, 127)
  line L19 (3.175, 114.3) -> (0, 114.3)
  line L20 (3.175, 12.7) -> (3.175, 0)
  line L21 (3.175, 190.5) -> (3.175, 177.8)
  line L22 (3.175, 177.8) -> (0, 177.8)
  line L23 (101.6, 50.8) -> (101.6, 38.1)
  line L24 (3.175, 50.8) -> (3.175, 38.1)
  line L25 (98.425, 152.4) -> (101.6, 152.4)
  line L26 (98.425, 50.8) -> (101.6, 50.8)
  line L27 (98.425, 152.4) -> (98.425, 139.7)
  line L28 (3.175, 139.7) -> (0, 139.7)
  line L29 (0, 139.7) -> (0, 127)
  line L30 (3.175, 101.6) -> (3.175, 88.9)
  line L31 (98.425, 101.6) -> (98.425, 95.25)
  line L32 (98.425, 203.2) -> (98.425, 190.5)
  line L33 (101.6, 152.4) -> (101.6, 139.7)
  line L34 (101.6, 203.2) -> (101.6, 190.5)
  line L35 (3.175, 203.2) -> (3.175, 190.5)
  line L36 (0, 0) -> (11.0998, 0)
  line L37 (98.425, 177.8) -> (98.425, 165.1)
  line L38 (98.425, 127) -> (98.425, 114.3)
  line L39 (0, 165.1) -> (0, 152.4)
  line L40 (11.0998, 0) -> (6.0198, 0)
  line L41 (98.425, 88.9) -> (98.425, 76.2)
  line L42 (0, 38.1) -> (3.175, 38.1)
  line L43 (98.425, 38.1) -> (98.425, 25.4)
  line L44 (101.6, 177.8) -> (101.6, 165.1)
  line L45 (98.425, 12.7) -> (101.6, 12.7)
  line L46 (0, 177.8) -> (0, 190.5)
  line L47 (98.425, 177.8) -> (101.6, 177.8)
  line L48 (0, 76.2) -> (0, 88.9)
  line L49 (0, 114.3) -> (0, 101.6)
  line L50 (3.175, 190.5) -> (0, 190.5)
  line L51 (98.425, 190.5) -> (101.6, 190.5)
  line L52 (101.6, 0) -> (0, 0)
  line L53 (98.425, 38.1) -> (101.6, 38.1)
  line L54 (90.5002, 0) -> (95.5802, 0)
  line L55 (3.175, 203.2) -> (101.6, 203.2)
  line L56 (98.425, 76.2) -> (101.6, 76.2)
  line L57 (98.425, 165.1) -> (101.6, 165.1)
  line L58 (98.425, 63.5) -> (98.425, 50.8)
  line L59 (98.425, 25.4) -> (101.6, 25.4)
  line L60 (0, 0) -> (0, 12.7)
  line L61 (3.175, 63.5) -> (0, 63.5)
  line L62 (98.425, 63.5) -> (101.6, 63.5)
  line L63 (0, 152.4) -> (0, 165.1)
  line L64 (0, 152.4) -> (3.175, 152.4)
  line L65 (0, 25.4) -> (0, 38.1)
  line L66 (0, 0) -> (12.065, 0)
  line L67 (3.175, 50.8) -> (0, 50.8)
  line L68 (101.6, 203.2) -> (98.425, 203.2)
  line L69 (98.425, 190.5) -> (98.425, 177.8)
  line L70 (101.6, 76.2) -> (101.6, 63.5)
  line L71 (101.6, 0) -> (90.5002, 0)
  line L72 (3.175, 25.4) -> (3.175, 12.7)
  line L73 (98.425, 25.4) -> (98.425, 12.7)
  line L74 (3.175, 38.1) -> (3.175, 25.4)
  line L75 (0, 12.7) -> (3.175, 12.7)
  line L76 (0, 50.8) -> (0, 63.5)
  line L77 (0, 25.4) -> (3.175, 25.4)
  line L78 (3.175, 177.8) -> (3.175, 165.1)
  line L79 (101.6, 0) -> (98.425, 0)
  line L80 (101.6, 0) -> (85.725, 0)
  line L81 (101.6, 25.4) -> (101.6, 12.7)
  line L82 (3.175, 76.2) -> (0, 76.2)
  line L83 (98.425, 165.1) -> (98.425, 152.4)
  line L84 (3.175, 63.5) -> (3.175, 50.8)
  line L85 (3.175, 152.4) -> (3.175, 139.7)
  line L86 (98.425, 76.2) -> (98.425, 63.5)
  line L87 (3.175, 165.1) -> (0, 165.1)
  line L88 (98.425, 50.8) -> (98.425, 38.1)
  line L89 (3.175, 76.2) -> (3.175, 63.5)
  line L90 (0, 0) -> (3.175, 0)
  line L91 (3.175, 88.9) -> (3.175, 76.2)
  line L92 (98.425, 203.2) -> (98.425, 177.8)
  line L93 (3.175, 0) -> (3.175, 59.055)
  line L94 (7.62, 139.7) -> (51.5837, 114.2474)
  line L95 (49.9801, 111.4777) -> (6.0165, 136.9303)
  line L96 (6.0165, 136.9303) -> (7.62, 139.7)
  line L97 (93.7411, 193.04) -> (49.7434, 167.6463)
  line L98 (92.1413, 195.8119) -> (93.7411, 193.04)
  line L99 (48.1436, 170.4182) -> (92.1413, 195.8119)
  line L100 (3.175, 60.2676) -> (4.1957, 60.2676)
  line L101 (4.1957, 60.2676) -> (6.35, 60.2676)
  line L102 (6.35, 60.2676) -> (95.8689, 92.8088)
  line L103 (94.7755, 95.8167) -> (5.2566, 63.2754)
  line L104 (49.9801, 111.4777) -> (50.2, 111.3504)
  line L105 (50.2, 111.3504) -> (51.8035, 114.1201)
  line L106 (51.8035, 114.1201) -> (51.5837, 114.2474)
  line L107 (95.8689, 92.8088) -> (96.1076, 92.8956)
  line L108 (96.1076, 92.8956) -> (95.0142, 95.9034)
  line L109 (95.0142, 95.9034) -> (94.7755, 95.8167)
  line L110 (49.7434, 167.6463) -> (49.5234, 167.5194)
  line L111 (49.5234, 167.5194) -> (47.9236, 170.2912)
  line L112 (47.9236, 170.2912) -> (48.1436, 170.4182)
  line L113 (5.2566, 63.2754) -> (6.35, 60.2676)
  dimension "d9" = 11.0998
  dimension "d10" = 11.0998
  dimension "d14" = 5.08
  dimension "d15" = 5.08
  dimension "d27" = 3.175
  dimension "d28" = 3.175
  dimension "d40" = 3.175
  dimension "d41" = 3.175
  dimension "d42" = 12.7
  dimension "d43" = 12.7
  dimension "d44" = 12.7
  dimension "d45" = 12.7
  dimension "d46" = 12.7
  dimension "d47" = 12.7
  dimension "d48" = 12.7
  dimension "d49" = 12.7
  dimension "d50" = 6.35
  dimension "d51" = 6.35
  dimension "d52" = 12.7
  dimension "d53" = 12.7
  dimension "d54" = 12.7
  dimension "d55" = 12.7
  dimension "d56" = 12.7
  dimension "d57" = 12.7
  dimension "d74" = 59.055
  dimension "d78" = 50.8
  dimension "d79" = 3.2004
  dimension "d80" = 50.8
  dimension "d81" = 50.8
  dimension "d82" = 3.2004
  dimension "d83" = 50.8
  dimension "d84" = 95.25
  dimension "d85" = 3.2004
  dimension "d86" = 95.25
  dimension "d87" = 0.254
  dimension "d88" = 0.254
  dimension "d89" = 3.2004
  dimension "d90" = 0.254
  dimension "d91" = 3.2004
  constraint coincident L36.start L52.end
  constraint vertical L60
  constraint perpendicular L55 L60
  constraint perpendicular L34 L55
  constraint perpendicular L52 L60
  constraint perpendicular L60 L66
  constraint perpendicular L34 L80
  constraint perpendicular L10 L34
  constraint coincident L54.start L52
  constraint perpendicular L36 L60
  constraint perpendicular L50 L60
  constraint perpendicular L21 L50
  constraint coincident L22.end L60
  constraint perpendicular L22 L60
  constraint perpendicular L22 L78
  constraint perpendicular L60 L87
  constraint collinear L46 L60
  constraint perpendicular L39 L87
  constraint perpendicular L39 L64
  constraint parallel L66 L90
  constraint perpendicular L14 L55
  constraint perpendicular L64 L85
  constraint perpendicular L28 L60
  constraint perpendicular L28 L29
  constraint coincident L4.end L14
  constraint perpendicular L4 L14
  constraint perpendicular L4 L16
  constraint perpendicular L16 L19
  constraint perpendicular L19 L49
  constraint midpoint L6.end L14
  constraint perpendicular L6 L14
  constraint perpendicular L6 L30
  constraint parallel L14 L91
  constraint parallel L14 L89
  constraint parallel L14 L84
  constraint parallel L14 L24
  constraint parallel L24 L74
  constraint parallel L14 L72
  constraint perpendicular L17 L60
  constraint coincident L48.start L60
  constraint perpendicular L60 L82
  constraint perpendicular L60 L61
  constraint coincident L67.end L60
  constraint perpendicular L60 L67
  constraint coincident L65.start L60
  constraint collinear L60 L63
  constraint collinear L2 L60
  constraint collinear L1 L60
  constraint collinear L48 L60
  constraint collinear L60 L76
  constraint collinear L60 L65
  constraint perpendicular L34 L68
  constraint perpendicular L34 L79
  constraint perpendicular L32 L55
  constraint perpendicular L34 L51
  constraint perpendicular L51 L69
  constraint coincident L44.start L34
  constraint perpendicular L34 L47
  constraint perpendicular L37 L47
  constraint coincident L44.end L34
  constraint perpendicular L34 L57
  constraint perpendicular L57 L83
  constraint coincident L25.end L34
  constraint perpendicular L25 L34
  constraint perpendicular L25 L27
  constraint coincident L0.end L34
  constraint perpendicular L0 L34
  constraint perpendicular L0 L18
  constraint coincident L11.end L34
  constraint perpendicular L11 L34
  constraint perpendicular L11 L38
  constraint coincident L3.end L34
  constraint perpendicular L3 L34
  constraint perpendicular L3 L8
  constraint perpendicular L12 L34
  constraint perpendicular L12 L31
  constraint parallel L7 L13
  constraint coincident L5.end L34
  constraint perpendicular L9 L34
  constraint perpendicular L9 L41
  constraint coincident L56.end L34
  constraint perpendicular L34 L56
  constraint perpendicular L56 L86
  constraint coincident L62.end L34
  constraint perpendicular L34 L62
  constraint perpendicular L58 L62
  constraint coincident L23.start L34
  constraint perpendicular L26 L34
  constraint perpendicular L26 L88
  constraint coincident L23.end L34
  constraint perpendicular L34 L53
  constraint perpendicular L43 L53
  constraint perpendicular L43 L59
  constraint perpendicular L59 L73
  constraint perpendicular L45 L73
  constraint collinear L34 L44
  constraint coincident L5.start L34
  constraint collinear L33 L44
  constraint collinear L15 L33
  constraint collinear L5 L15
  constraint collinear L5 L70
  constraint collinear L23 L70
  constraint collinear L23 L81
  constraint coincident L84 L93.end
  constraint coincident L84 L100.start
  constraint perpendicular L84 L100
  constraint perpendicular L93 L101
  constraint perpendicular L95 L105
  constraint parallel L102 L107
  constraint perpendicular L107 L108
  constraint parallel L97 L110
  constraint perpendicular L110 L111
  constraint perpendicular L111 L112
  constraint perpendicular L102 L113
  measures "d9" distance of L10.start L54.start
  measures "d10" distance of L36.start L36.end
  measures "d14" distance of L36.end L40.end
  measures "d15" distance of L54.end L54.start
  measures "d27" distance of L39.end L64.end
  measures "d28" distance of L36.start L14.start
  measures "d40" distance of L7.end L34.start
  measures "d41" distance of L7.start L10.start
  measures "d42" distance of L7.end L32.end
  measures "d43" distance of L32.end L37.start
  measures "d44" distance of L37.end L37.start
  measures "d45" distance of L25.start L37.end
  measures "d46" distance of L0.start L25.start
  measures "d47" distance of L0.start L11.start
  measures "d48" distance of L3.start L11.start
  measures "d49" distance of L8.end L3.start
  measures "d50" distance of L8.end L13.start
  measures "d51" distance of L13.start L9.start
  measures "d52" distance of L9.start L41.end
  measures "d53" distance of L41.end L58.start
  measures "d54" distance of L58.start L26.start
  measures "d55" distance of L26.start L43.start
  measures "d56" distance of L43.end L43.start
  measures "d57" distance of L43.end L45.start
  measures "d74" distance of L14.start L93.end
  measures "d78" distance of L94.start L94.end
  measures "d79" distance of L95.start L94.end
  measures "d80" distance of L95.start L95.end
  measures "d81" distance of L97.start L97.end
  measures "d82" distance of L99.start L97.end
  measures "d83" distance of L98.start L99.start
  measures "d84" distance of L101.end L102.end
  measures "d85" distance of L102.end L103.start
  measures "d86" distance of L103.start L103.end
  measures "d87" distance of L95.start L104.end
  measures "d88" distance of L102.end L107.end
  measures "d89" distance of L107.end L108.end
  measures "d90" distance of L97.end L110.end
  measures "d91" distance of L110.end L111.end
extrude "Extrude1" add sketch "Sketch1" along normal blind 3.175
sketch "Sketch2" plane through (0, 0, 0) normal (1, 0, 0) x (0, 1, 0)
equation "d9 = 0.5 in - 0.063 in"

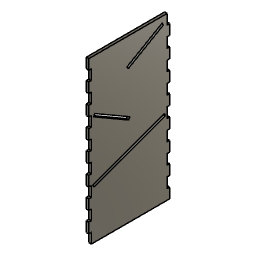
design "Dice Tower (Left Side)"
Autodesk Fusion 360 part; units mm, degrees
sketch "Sketch1" plane through (0, 0, 0) normal (1, 0, 0) x (0, 1, 0)
  line L0 (-98.425, 88.9) -> (-101.6, 88.9)
  line L1 (-98.425, 38.1) -> (-98.425, 25.4)
  line L2 (-98.425, 76.2) -> (-101.6, 76.2)
  line L3 (-101.6, 0) -> (-100.0125, 0)
  line L4 (-98.425, 190.5) -> (-98.425, 177.8)
  line L5 (-101.6, 203.2) -> (-98.425, 203.2)
  line L6 (-98.425, 177.8) -> (-98.425, 165.1)
  line L7 (-98.425, 203.2) -> (-98.425, 177.8)
  line L8 (-3.175, 177.8) -> (0, 177.8)
  line L9 (-98.425, 127) -> (-101.6, 127)
  line L10 (-3.175, 165.1) -> (0, 165.1)
  line L11 (-98.425, 165.1) -> (-98.425, 152.4)
  line L12 (0, 12.7) -> (-3.175, 12.7)
  line L13 (0, 127) -> (-3.175, 127)
  line L14 (-101.6, 76.2) -> (-101.6, 63.5)
  line L15 (-98.425, 63.5) -> (-98.425, 50.8)
  line L16 (-98.425, 114.3) -> (-98.425, 101.6)
  line L17 (-101.6, 101.6) -> (-101.6, 88.9)
  line L18 (-101.6, 0) -> (-98.425, 0)
  line L19 (-98.425, 63.5) -> (-101.6, 63.5)
  line L20 (-101.6, 0) -> (-90.5002, 0)
  line L21 (-3.175, 190.5) -> (-3.175, 177.8)
  line L22 (-3.175, 50.8) -> (0, 50.8)
  line L23 (0, 25.4) -> (-3.175, 25.4)
  line L24 (-3.175, 152.4) -> (-3.175, 139.7)
  line L25 (0, 38.1) -> (-3.175, 38.1)
  line L26 (-101.6, 177.8) -> (-101.6, 165.1)
  line L27 (0, 0) -> (-3.175, 0)
  line L28 (-3.175, 190.5) -> (0, 190.5)
  line L29 (-3.175, 50.8) -> (-3.175, 38.1)
  line L30 (-101.6, 203.2) -> (-101.6, 190.5)
  line L31 (-101.6, 127) -> (-101.6, 114.3)
  line L32 (-98.425, 114.3) -> (-101.6, 114.3)
  line L33 (0, 0) -> (-11.0998, 0)
  line L34 (-98.425, 139.7) -> (-98.425, 127)
  line L35 (-3.175, 177.8) -> (-3.175, 165.1)
  line L36 (-98.425, 165.1) -> (-101.6, 165.1)
  line L37 (-11.0998, 0) -> (-6.0198, 0)
  line L38 (0, 152.4) -> (-3.175, 152.4)
  line L39 (0, 0) -> (-12.065, 0)
  line L40 (-3.175, 76.2) -> (-3.175, 63.5)
  line L41 (-3.175, 139.7) -> (0, 139.7)
  line L42 (-3.175, 12.7) -> (-3.175, 0)
  line L43 (-90.5002, 0) -> (-95.5802, 0)
  line L44 (-98.425, 101.6) -> (-101.6, 101.6)
  line L45 (-3.175, 101.6) -> (-3.175, 88.9)
  line L46 (-3.175, 0) -> (-3.175, 59.055)
  line L47 (-3.175, 88.9) -> (-3.175, 76.2)
  line L48 (-98.425, 177.8) -> (-101.6, 177.8)
  line L49 (-3.175, 38.1) -> (-3.175, 25.4)
  line L50 (-98.425, 152.4) -> (-98.425, 139.7)
  line L51 (-98.425, 203.2) -> (-98.425, 190.5)
  line L52 (-98.425, 139.7) -> (-101.6, 139.7)
  line L53 (-3.175, 63.5) -> (0, 63.5)
  line L54 (-3.175, 203.2) -> (-3.175, 190.5)
  line L55 (-98.425, 127) -> (-98.425, 114.3)
  line L56 (-3.175, 63.5) -> (-3.175, 50.8)
  line L57 (-3.175, 88.9) -> (0, 88.9)
  line L58 (-3.175, 114.3) -> (0, 114.3)
  line L59 (0, 101.6) -> (-3.175, 101.6)
  line L60 (-3.175, 127) -> (-3.175, 114.3)
  line L61 (-98.425, 190.5) -> (-101.6, 190.5)
  line L62 (-98.425, 0) -> (-98.425, 203.2)
  line L63 (-3.175, 76.2) -> (0, 76.2)
  line L64 (-98.425, 152.4) -> (-101.6, 152.4)
  line L65 (-98.425, 25.4) -> (-98.425, 12.7)
  line L66 (-101.6, 152.4) -> (-101.6, 139.7)
  line L67 (-98.425, 38.1) -> (-101.6, 38.1)
  line L68 (-101.6, 0) -> (0, 0)
  line L69 (-98.425, 50.8) -> (-101.6, 50.8)
  line L70 (-101.6, 50.8) -> (-101.6, 38.1)
  line L71 (-98.425, 50.8) -> (-98.425, 38.1)
  line L72 (-101.6, 0) -> (-85.725, 0)
  line L73 (-3.175, 0) -> (-3.175, 203.2)
  line L74 (-98.425, 101.6) -> (-98.425, 95.25)
  line L75 (-98.425, 95.25) -> (-98.425, 88.9)
  line L76 (-3.175, 203.2) -> (-101.6, 203.2)
  line L77 (-98.425, 88.9) -> (-98.425, 76.2)
  line L78 (-3.175, 25.4) -> (-3.175, 12.7)
  line L79 (-98.425, 76.2) -> (-98.425, 63.5)
  line L80 (-101.6, 25.4) -> (-101.6, 12.7)
  line L81 (-98.425, 12.7) -> (-101.6, 12.7)
  line L82 (-98.425, 25.4) -> (-101.6, 25.4)
  line L83 (-6.8245, 95.8167) -> (-96.3434, 63.2754)
  line L84 (-53.6764, 170.2912) -> (-53.4564, 170.4182)
  line L85 (-6.5858, 95.9034) -> (-6.8245, 95.8167)
  line L86 (-51.6199, 111.4777) -> (-51.4, 111.3504)
  line L87 (-7.8589, 193.04) -> (-51.8566, 167.6463)
  line L88 (-95.5835, 136.9303) -> (-93.98, 139.7)
  line L89 (-9.4587, 195.8119) -> (-7.8589, 193.04)
  line L90 (-51.8566, 167.6463) -> (-52.0766, 167.5194)
  line L91 (-5.4924, 92.8956) -> (-6.5858, 95.9034)
  line L92 (-51.6199, 111.4777) -> (-95.5835, 136.9303)
  line L93 (-93.98, 139.7) -> (-50.0163, 114.2474)
  line L94 (-96.3434, 63.2754) -> (-95.25, 60.2676)
  line L95 (-53.4564, 170.4182) -> (-9.4587, 195.8119)
  line L96 (-5.7311, 92.8088) -> (-5.4924, 92.8956)
  line L97 (-51.4, 111.3504) -> (-49.7965, 114.1201)
  line L98 (-95.25, 60.2676) -> (-5.7311, 92.8088)
  line L99 (-49.7965, 114.1201) -> (-50.0163, 114.2474)
  line L100 (-52.0766, 167.5194) -> (-53.6764, 170.2912)
  line L101 (0, 190.5) -> (0, 177.8)
  line L102 (0, 165.1) -> (0, 152.4)
  line L103 (0, 139.7) -> (0, 127)
  line L104 (0, 114.3) -> (0, 101.6)
  line L105 (0, 88.9) -> (0, 76.2)
  line L106 (0, 63.5) -> (0, 50.8)
  line L107 (0, 38.1) -> (0, 25.4)
  line L108 (0, 12.7) -> (0, 0)
  dimension "d92" = 50.8
  dimension "d93" = 3.2004
  dimension "d94" = 50.8
  dimension "d95" = 50.8
  dimension "d96" = 3.2004
  dimension "d97" = 50.8
  dimension "d98" = 95.25
  dimension "d99" = 3.2004
  dimension "d100" = 95.25
  dimension "d101" = 0.254
  dimension "d102" = 0.254
  dimension "d103" = 3.2004
  dimension "d104" = 0.254
  dimension "d105" = 3.2004
  constraint perpendicular L92 L97
  constraint parallel L96 L98
  constraint perpendicular L91 L96
  constraint parallel L87 L90
  constraint perpendicular L90 L100
  constraint perpendicular L84 L100
  constraint perpendicular L94 L98
  constraint perpendicular L8 L101
  constraint perpendicular L38 L102
  constraint perpendicular L13 L103
  constraint perpendicular L59 L104
  constraint perpendicular L63 L105
  constraint perpendicular L22 L106
  constraint parallel L106 L107
  constraint perpendicular L27 L108
  measures "d92" distance of L88.end L93.end
  measures "d93" distance of L93.end L86.start
  measures "d94" distance of L88.start L86.start
  measures "d95" distance of L87.start L87.end
  measures "d96" distance of L84.end L87.end
  measures "d97" distance of L84.end L89.start
  measures "d98" distance of L94.end L96.start
  measures "d99" distance of L96.start L83.start
  measures "d100" distance of L83.end L83.start
  measures "d101" distance of L86.start L86.end
  measures "d102" distance of L96.start L91.start
  measures "d103" distance of L85.start L91.start
  measures "d104" distance of L90.end L87.end
  measures "d105" distance of L84.start L90.end
extrude "Extrude1" add sketch "Sketch1" along normal blind 3.175
sketch "Sketch2" plane through (0, 0, 0) normal (1, 0, 0) x (0, 1, 0)
